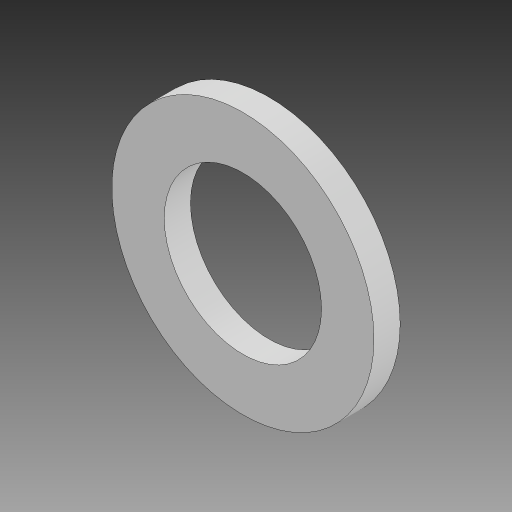
# Autodesk Inventor part: support-ring
Saved by Autodesk Inventor 2023 (Build 270158000, 158)
## iProperties
Created: 2024-01-30
Part Number: support-ring
Material: Všeobecné
Document SubType Name: Modeling
Designer: matej
Mass: 0.0502655 g
Surface Area: 1.50796 cm^2
Volume: 0.0502655 cm^3
Density: 1 g/cm^3
Appearance: Výchozí
Author: matej
## iProperties of the stored document support-ring_3D tisk.ipt
Created: 2024-01-30
Part Number: support-ring_3D tisk
Material: Všeobecné
Document SubType Name: Modeling
Designer: matej
Mass: 0.0290283 g
Surface Area: 0.995257 cm^2
Volume: 0.0290283 cm^3
Density: 1 g/cm^3
Appearance: Výchozí
Author: matej
Autodesk Inventor part; units mm, degrees
ref_plane "YZ Plane" through (0, 0, 0) normal (1, 0, 0) x (0, 1, 0)
ref_plane "XZ Plane" through (0, 0, 0) normal (0, 1, 0) x (-1, 0, 0)
ref_plane "XY Plane" through (0, 0, 0) normal (0, 0, 1) x (1, 0, 0)
sketch "Náčrt1" plane through (0, 0, 0) normal (0, 0, 1) x (1, 0, 0)
  circle A0 centre (0, 0) radius 3
  circle A1 centre (0, 0) radius 5
  dimension "d0" = 6
  dimension "d1" = 10
  constraints: 2 centre point, 2 coincident
  measures "d0" diameter of A0
  measures "d1" diameter of A1
extrude "Vysunutí1" add sketch "Náčrt1" along normal blind 1
